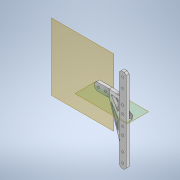
# Autodesk Inventor part: body_linker_2_8d
Saved by Autodesk Inventor 2023 (Build 270158000, 158)
## iProperties
Created: 2021-03-15
Part Number: body_linker_2_8d
Material: Generic
Document SubType Name: Modeling
Designer: Shuang Peng
Density: 1 g/cm^3
Appearance: Default
Author: Shuang Peng
Autodesk Inventor part; units mm, degrees
ref_plane "YZ Plane" through (0, 0, 0) normal (1, 0, 0) x (0, 1, 0)
ref_plane "XZ Plane" through (0, 0, 0) normal (0, 1, 0) x (-1, 0, 0)
ref_plane "XY Plane" through (0, 0, 0) normal (0, 0, 1) x (1, 0, 0)
sketch "Sketch1" plane through (0, 0, 0) normal (0, 0, 1) x (1, 0, 0)
  circle A0 centre (-13.3324, -4) radius 1.6 projected
  circle A1 centre (-13.3324, -14) radius 1.6 projected
  line L0 (-25.6648, -6) -> (-20.718, -6) projected
  arc A2 (-19.718, -7) -> (-20.718, -6) centre (-20.718, -7) ccw projected
  line L1 (-19.718, -7) -> (-19.718, -11) projected
  arc A3 (-20.718, -12) -> (-19.718, -11) centre (-20.718, -11) ccw projected
  line L2 (-20.718, -12) -> (-25.6648, -12) projected
  arc A4 (-26.6648, -11) -> (-25.6648, -12) centre (-25.6648, -11) ccw projected
  line L3 (-26.6648, -11) -> (-26.6648, -19) projected
  line L4 (-26.6648, -19) -> (0, -19) projected
  line L5 (0, -11) -> (0, -19) projected
  arc A5 (-1, -12) -> (0, -11) centre (-1, -11) ccw projected
  line L6 (-1, -12) -> (-5.9469, -12) projected
  arc A6 (-6.9469, -11) -> (-5.9469, -12) centre (-5.9469, -11) ccw projected
  line L7 (-6.9469, -11) -> (-6.9469, -7) projected
  arc A7 (-5.9469, -6) -> (-6.9469, -7) centre (-5.9469, -7) ccw projected
  line L8 (-5.9469, -6) -> (-1, -6) projected
  arc A8 (0, -7) -> (-1, -6) centre (-1, -7) ccw projected
  line L9 (0, 1) -> (0, -7) projected
  line L10 (-26.6648, 1) -> (0, 1) projected
  line L11 (-26.6648, 1) -> (-26.6648, -7) projected
  arc A9 (-25.6648, -6) -> (-26.6648, -7) centre (-25.6648, -7) ccw projected
  circle A10 centre (-13.3324, 53) radius 1.6 projected
  circle A11 centre (-13.3324, 63) radius 1.6 projected
  line L12 (-25.6648, 55) -> (-20.718, 55) projected
  arc A12 (-26.6648, 56) -> (-25.6648, 55) centre (-25.6648, 56) ccw projected
  line L13 (-26.6648, 48) -> (-26.6648, 56) projected
  line L14 (-26.6648, 48) -> (0, 48) projected
  line L15 (0, 48) -> (0, 56) projected
  arc A13 (-1, 55) -> (0, 56) centre (-1, 56) ccw projected
  line L16 (-5.9469, 55) -> (-1, 55) projected
  arc A14 (-6.9469, 56) -> (-5.9469, 55) centre (-5.9469, 56) ccw projected
  line L17 (-6.9469, 60) -> (-6.9469, 56) projected
  arc A15 (-5.9469, 61) -> (-6.9469, 60) centre (-5.9469, 60) ccw projected
  line L18 (-1, 61) -> (-5.9469, 61) projected
  arc A16 (0, 60) -> (-1, 61) centre (-1, 60) ccw projected
  line L19 (0, 60) -> (0, 68) projected
  line L20 (-26.6648, 68) -> (0, 68) projected
  line L21 (-26.6648, 60) -> (-26.6648, 68) projected
  arc A17 (-25.6648, 61) -> (-26.6648, 60) centre (-25.6648, 60) ccw projected
  line L22 (-20.718, 61) -> (-25.6648, 61) projected
  arc A18 (-19.718, 60) -> (-20.718, 61) centre (-20.718, 60) ccw projected
  line L23 (-19.718, 56) -> (-19.718, 60) projected
  arc A19 (-20.718, 55) -> (-19.718, 56) centre (-20.718, 56) ccw projected
  line L24 (-13.3324, 53) -> (-13.3324, -4)
  line L25 (-9.8324, -19) -> (-16.8324, -19)
  line L26 (-16.8324, -19) -> (-16.8324, 68)
  line L27 (-16.8324, 68) -> (-9.8324, 68)
  line L28 (-9.8324, 68) -> (-9.8324, -19)
  line L29 (-9.8324, -19) -> (-16.8324, 68) construction
  line L30 (-16.8324, -19) -> (-9.8324, 68) construction
  circle A20 centre (-13.3324, -14) radius 1
  circle A21 centre (-13.3324, -4) radius 1
  circle A22 centre (-13.3324, 53) radius 1
  circle A23 centre (-13.3324, 63) radius 1
  point P0 (0, 0)
  point P1 (-13.3324, 24.5)
  dimension "d0" = 7
  dimension "d1" = 87
  dimension "d2" = 2
  dimension "d3" = 2
  dimension "d4" = 2
  dimension "d5" = 2
  constraints: 14 end point, 4 centre point, 4 coincident, 3 midpoint, 2 parallel, 1 horizontal, 1 perpendicular, 1 vertical
  measures "d0" distance of L25.start L25.end
  measures "d1" distance of L25.end L26.end
  measures "d2" diameter of A20
  measures "d3" diameter of A21
  measures "d4" diameter of A22
  measures "d5" diameter of A23
extrude "Extrusion1" add sketch "Sketch1" along normal blind 3 contours A0 | A1 | L26 L14 L24 L10 | L10 L28 L4 L26 | L24 L14 L28 L10 | L26 L20 L28 L14 | A10 | A11
ref_plane "Work Plane1" through (-45.4275, 48, -16.9065) normal (0, 0, 1) x (1, 0, 0)
ref_plane "Work Plane2" through (-45.4275, 48, -16.9065) normal (0, 0, 1) x (1, 0, 0)
sketch "Sketch2" plane through (-45.4275, 48, -16.9065) normal (0, 0, 1) x (1, 0, 0)
  circle A0 centre (-48.7456, -23.5) radius 1.5 projected
  circle A1 centre (-9.8354, -23.5) radius 1.5 projected
  circle A2 centre (-55.7456, -23.5) radius 1.5 projected
  circle A3 centre (-2.8354, -23.5) radius 1.5 projected
  line L0 (0, 8) -> (0, -55) projected
  line L1 (0, 8) -> (-2.7967, 8) projected
  line L2 (-2.7967, 8) -> (-15.1567, 2.005) projected
  arc A4 (-23.8848, 0) -> (-15.1567, 2.005) centre (-23.8848, 20) ccw projected
  line L3 (-23.8848, 0) -> (-34.6962, 0) projected
  arc A5 (-43.4243, 2.005) -> (-34.6962, 0) centre (-34.6962, 20) ccw projected
  line L4 (-43.4243, 2.005) -> (-55.7843, 8) projected
  line L5 (-55.7843, 8) -> (-58.581, 8) projected
  line L6 (-58.581, 8) -> (-58.581, -55) projected
  line L7 (-58.581, -55) -> (-55.7843, -55) projected
  line L8 (-55.7843, -55) -> (-43.4243, -49.005) projected
  arc A6 (-34.6962, -47) -> (-43.4243, -49.005) centre (-34.6962, -67) ccw projected
  line L9 (-23.8848, -47) -> (-34.6962, -47) projected
  arc A7 (-15.1567, -49.005) -> (-23.8848, -47) centre (-23.8848, -67) ccw projected
  line L10 (-15.1567, -49.005) -> (-2.7967, -55) projected
  line L11 (-2.7967, -55) -> (0, -55) projected
  line L12 (-2.8354, -23.5) -> (-9.8354, -23.5)
  line L13 (-13.8354, -27.5) -> (-13.8354, -19.5)
  line L14 (-13.8354, -19.5) -> (1.1646, -19.5)
  line L15 (1.1646, -19.5) -> (1.1646, -27.5)
  line L16 (1.1646, -27.5) -> (-13.8354, -27.5)
  line L17 (-13.8354, -27.5) -> (1.1646, -19.5) construction
  line L18 (-13.8354, -19.5) -> (1.1646, -27.5) construction
  circle A8 centre (-2.8354, -23.5) radius 1
  circle A9 centre (-9.8354, -23.5) radius 1
  circle A10 centre (-36.7456, -23.5) radius 1.5 projected
  circle A11 centre (-21.8354, -23.5) radius 1.5 projected
  line L19 (-18.1506, -17.698) -> (-8.4396, -10.4664) projected
  arc A12 (-6.5914, -10.1803) -> (-8.4396, -10.4664) centre (-7.2451, -12.0705) ccw projected
  line L20 (-6.5914, -10.1803) -> (-4.1818, -11.0136) projected
  arc A13 (-2.8354, -12.9037) -> (-4.1818, -11.0136) centre (-4.8354, -12.9037) ccw projected
  line L21 (-2.8354, -12.9037) -> (-2.8354, -17.5) projected
  arc A14 (-4.8354, -19.5) -> (-2.8354, -17.5) centre (-4.8354, -17.5) ccw projected
  line L22 (-4.8354, -19.5) -> (-17.5533, -19.5) projected
  arc A15 (-18.1506, -17.698) -> (-17.5533, -19.5) centre (-17.5533, -18.5) ccw projected
  line L23 (-50.1414, -10.4664) -> (-40.4304, -17.698) projected
  arc A16 (-41.0277, -19.5) -> (-40.4304, -17.698) centre (-41.0277, -18.5) ccw projected
  line L24 (-41.0277, -19.5) -> (-53.7456, -19.5) projected
  arc A17 (-55.7456, -17.5) -> (-53.7456, -19.5) centre (-53.7456, -17.5) ccw projected
  line L25 (-55.7456, -17.5) -> (-55.7456, -12.9037) projected
  arc A18 (-54.3992, -11.0136) -> (-55.7456, -12.9037) centre (-53.7456, -12.9037) ccw projected
  line L26 (-54.3992, -11.0136) -> (-51.9896, -10.1803) projected
  arc A19 (-50.1414, -10.4664) -> (-51.9896, -10.1803) centre (-51.3359, -12.0705) ccw projected
  line L27 (-8.4396, -36.5336) -> (-18.1506, -29.302) projected
  arc A20 (-17.5533, -27.5) -> (-18.1506, -29.302) centre (-17.5533, -28.5) ccw projected
  line L28 (-17.5533, -27.5) -> (-4.8354, -27.5) projected
  arc A21 (-2.8354, -29.5) -> (-4.8354, -27.5) centre (-4.8354, -29.5) ccw projected
  line L29 (-2.8354, -29.5) -> (-2.8354, -34.0963) projected
  arc A22 (-4.1818, -35.9864) -> (-2.8354, -34.0963) centre (-4.8354, -34.0963) ccw projected
  line L30 (-4.1818, -35.9864) -> (-6.5914, -36.8197) projected
  arc A23 (-8.4396, -36.5336) -> (-6.5914, -36.8197) centre (-7.2451, -34.9295) ccw projected
  line L31 (-40.4304, -29.302) -> (-50.1414, -36.5336) projected
  arc A24 (-51.9896, -36.8197) -> (-50.1414, -36.5336) centre (-51.3359, -34.9295) ccw projected
  line L32 (-51.9896, -36.8197) -> (-54.3992, -35.9864) projected
  arc A25 (-55.7456, -34.0963) -> (-54.3992, -35.9864) centre (-53.7456, -34.0963) ccw projected
  line L33 (-55.7456, -34.0963) -> (-55.7456, -29.5) projected
  arc A26 (-53.7456, -27.5) -> (-55.7456, -29.5) centre (-53.7456, -29.5) ccw projected
  line L34 (-53.7456, -27.5) -> (-41.0277, -27.5) projected
  arc A27 (-40.4304, -29.302) -> (-41.0277, -27.5) centre (-41.0277, -28.5) ccw projected
  arc A28 (-11.559, -7.802) -> (-12.1562, -6) centre (-12.1562, -7) ccw projected
  line L35 (-11.559, -7.802) -> (-28.096, -20.1168) projected
  arc A29 (-30.485, -20.1168) -> (-28.096, -20.1168) centre (-29.2905, -18.5127) ccw projected
  line L36 (-30.485, -20.1168) -> (-47.022, -7.802) projected
  arc A30 (-46.4248, -6) -> (-47.022, -7.802) centre (-46.4248, -7) ccw projected
  line L37 (-46.4248, -6) -> (-12.1562, -6) projected
  arc A31 (-12.1562, -41) -> (-11.559, -39.198) centre (-12.1562, -40) ccw projected
  line L38 (-12.1562, -41) -> (-46.4248, -41) projected
  arc A32 (-47.022, -39.198) -> (-46.4248, -41) centre (-46.4248, -40) ccw projected
  line L39 (-47.022, -39.198) -> (-30.485, -26.8832) projected
  arc A33 (-28.096, -26.8832) -> (-30.485, -26.8832) centre (-29.2905, -28.4873) ccw projected
  line L40 (-28.096, -26.8832) -> (-11.559, -39.198) projected
  circle A34 centre (-52.7905, -6) radius 1.5 projected
  circle A35 centre (-5.7905, -6) radius 1.5 projected
  circle A36 centre (-52.7905, -41) radius 1.5 projected
  circle A37 centre (-5.7905, -41) radius 1.5 projected
  point P0 (45.4275, -48)
  point P1 (-6.3354, -23.5)
  dimension "d8" = 8
  dimension "d9" = 15
  dimension "d10" = 2
  dimension "d11" = 2
  constraints: 14 end point, 3 midpoint, 2 centre point, 2 coincident, 2 parallel, 1 horizontal, 1 perpendicular, 1 vertical
  measures "d8" distance of L13.start L13.end
  measures "d9" distance of L13.end L14.end
  measures "d10" diameter of A8
  measures "d11" diameter of A9
extrude "Extrusion2" add sketch "Sketch2" along normal blind 3 contours A1 | A3 | L14 L15 L16 L0 | L0 L16 L13 L14
sketch "Sketch3" plane through (-16.8324, -19, 0) normal (-1, 0, 0) x (0, 0, 1)
  line L0 (0, 87) -> (0, 0) projected
  line L1 (0, 0) -> (3, 0) projected
  line L2 (3, 87) -> (3, 0) projected
  line L3 (0, 87) -> (3, 87) projected
  line L4 (0, 87) -> (0, 0) projected
  line L5 (0, 43.5) -> (3, 43.5)
  line L6 (3, 43.5) -> (0, 43.5)
  line L7 (0, 43.5) -> (0, 23.5)
  line L8 (0, 23.5) -> (3, 23.5)
  line L9 (3, 23.5) -> (3, 43.5)
  line L10 (0, 43.5) -> (3, 43.5)
  line L11 (3, 43.5) -> (3, 63.5)
  line L12 (3, 63.5) -> (0, 63.5)
  line L13 (0, 63.5) -> (0, 43.5)
  point P0 (0, 19)
  dimension "d14" = 3
  dimension "d15" = 20
  dimension "d16" = 3
  dimension "d17" = 20
  constraints: 18 end point, 4 parallel, 2 horizontal, 2 midpoint, 2 perpendicular
  measures "d14" distance of L8.end L7.end
  measures "d15" distance of L7.end L6.end
  measures "d16" distance of L12.end L11.end
  measures "d17" distance of L11.end L10.end
loft "Loft1" add profiles "Sketch3" section 2 edges at (-44.2629, 24.5, -16.9065) (-44.2629, 28.5, -15.4065) (-44.2629, 24.5, -13.9065) (-44.2629, 20.5, -15.4065) contours L12 L2 L5 L0 | L5 L2 L8 L0
ref_plane "Work Plane3" through (-59.2629, 24.5, -16.9065) normal (0, -1, 0) x (1, 0, 0)
sketch "Sketch5" plane through (-59.2629, 24.5, -16.9065) normal (0, -1, 0) x (1, 0, 0)
  line L0 (42.4305, 19.9065) -> (42.4305, 16.9065) projected
  line L1 (42.4305, 19.9065) -> (15, 3) projected
  line L2 (15, 0) -> (15, 3) projected
  line L3 (42.4305, 16.9065) -> (15, 0) projected
  line L4 (42.4305, 16.9065) -> (49.4305, 16.9065) projected
  line L5 (49.4305, 16.9065) -> (49.4305, 19.9065) projected
  line L6 (42.4305, 19.9065) -> (49.4305, 19.9065) projected
  line L7 (42.4305, 16.9065) -> (42.4305, 19.9065) projected
  line L8 (49.4305, 16.9065) -> (49.4305, 11.9065)
  line L9 (49.4305, 11.9065) -> (15, 0)
  point P0 (59.2629, 16.9065)
  point P1 (42.4305, 16.9065)
  dimension "d22" = 5
  constraints: 4 end point, 1 vertical
  measures "d22" distance of L4.end L8.end
extrude "Extrusion3" add sketch "Sketch5" against normal mid plane 2 contours L4 L8 L9 L3
fillet "Fillet1" radius 3 1 edges at (-9.8324, 24.5, -5)
sketch "Sketch6" plane through (-16.8324, 25.5, 0) normal (0.5246872, 0, -0.8512951) x (-0.8512951, 0, -0.5246872)
  line L0 (0, 0) -> (32.222, 0) projected
  line L1 (32.222, 0) -> (32.222, 3) projected
  line L2 (0, 19) -> (32.222, 3) projected
  line L3 (0, 19) -> (0, 0) projected
  line L4 (32.222, -2) -> (0, -2) projected
  line L5 (0, -2) -> (0, -21) projected
  line L6 (0, -21) -> (32.222, -5) projected
  line L7 (32.222, -5) -> (32.222, -2) projected
  line L8 (2, 13.5409) -> (2, 2)
  line L9 (2, 2) -> (25.242, 2)
  line L10 (25.242, 2) -> (2, 13.5409)
  line L11 (2, -4) -> (2, -15.5409)
  line L12 (2, -15.5409) -> (25.242, -4)
  line L13 (25.242, -4) -> (2, -4)
  line L14 (-1.25, 0) -> (32.222, 0) projected
  line L15 (32.222, -2) -> (-1.25, -2) projected
  point P0 (-14.3294, -25.5)
  dimension "d26" = 2
  dimension "d27" = 2
  dimension "d28" = 4
  dimension "d29" = 4
  dimension "d30" = 2
  dimension "d31" = 2
  constraints: 12 end point, 6 parallel, 1 horizontal
  measures "d26" distance between parallel lines of L3 L8
  measures "d27" distance between parallel lines of L14 L9
  measures "d28" distance between parallel lines of L2 L10
  measures "d29" distance between parallel lines of L6 L12
  measures "d30" distance between parallel lines of L4 L13
  measures "d31" distance between parallel lines of L5 L11
extrude "Extrusion4" cut sketch "Sketch6" against normal blind 3 contours L10 L9 L8 | L13 L12 L11
fillet "Fillet2" radius 0.5 2 edges at (-38.9908, 27.5, -12.1571) (-38.9908, 21.5, -12.1571)
fillet "Fillet2" radius 1 2 edges at (-19.205, 39.0409, 0.0377) (-19.205, 9.9591, 0.0377)
fillet "Fillet2" radius 1.5 2 edges at (-19.205, 27.5, 0.0377) (-19.205, 21.5, 0.0377)
fillet "Fillet3" radius 3 2 edges at (-16.8324, 44.5, 1.5) (-16.8324, 4.5, 1.5)
chamfer "Chamfer1" distance 2 angle 45 4 edges at (-16.8324, 68, 1.5) (-9.8324, 68, 1.5) (-16.8324, -19, 1.5) (-9.8324, -19, 1.5)
chamfer "Chamfer2" distance 2 angle 45 2 edges at (-59.2629, 20.5, -15.4065) (-59.2629, 28.5, -15.4065)
sketch "Sketch7" plane through (0, 0, 0) normal (0, 0, -1) x (-1, 0, 0)
  line L0 (11.8324, -19) -> (9.8324, -17) projected
  line L1 (14.8324, -19) -> (11.8324, -19) projected
  line L2 (16.8324, -17) -> (14.8324, -19) projected
  line L3 (16.8324, 2.7768) -> (16.8324, -17) projected
  line L4 (16.8324, 23.5) -> (16.8324, 2.7768) projected
  line L5 (16.8324, 23.5) -> (9.8324, 23.5) projected
  line L6 (9.8324, -17) -> (9.8324, 23.5) projected
  circle A0 centre (13.3324, -4) radius 1 projected
  circle A1 centre (13.3324, -14) radius 1 projected
  circle A2 centre (13.3324, 53) radius 1 projected
  circle A3 centre (13.3324, 63) radius 1 projected
  line L7 (9.8324, 66) -> (11.8324, 68) projected
  line L8 (9.8324, 25.5) -> (9.8324, 66) projected
  line L9 (9.8324, 25.5) -> (16.8324, 25.5) projected
  line L10 (16.8324, 46.2232) -> (16.8324, 25.5) projected
  line L11 (16.8324, 66) -> (16.8324, 46.2232) projected
  line L12 (14.8324, 68) -> (16.8324, 66) projected
  line L13 (11.8324, 68) -> (14.8324, 68) projected
  line L14 (16.8324, 23.5) -> (9.8324, 23.5)
  circle A4 centre (13.3324, -4) radius 1 projected
  line L15 (13.3324, -4) -> (13.3324, 11)
  line L16 (13.3324, 11) -> (13.3324, 19)
  circle A5 centre (13.3324, 53) radius 1 projected
  line L17 (13.3324, 53) -> (13.3324, 38)
  line L18 (13.3324, 38) -> (13.3324, 30)
  circle A6 centre (13.3324, 11) radius 1
  circle A7 centre (13.3324, 19) radius 1
  circle A8 centre (13.3324, 30) radius 1
  circle A9 centre (13.3324, 38) radius 1
  point P0 (0, 0)
  dimension "d44" = 15
  dimension "d45" = 8
  dimension "d46" = 15
  dimension "d47" = 8
  dimension "d48" = 2
  dimension "d49" = 2
  dimension "d50" = 2
  dimension "d51" = 2
  constraints: 10 end point, 4 centre point, 4 coincident, 3 vertical, 1 collinear, 1 point on line
  measures "d44" distance of L15.start L15.end
  measures "d45" distance of L15.end L16.end
  measures "d46" distance of L17.start L17.end
  measures "d47" distance of L17.end L18.end
  measures "d48" diameter of A6
  measures "d49" diameter of A7
  measures "d50" diameter of A8
  measures "d51" diameter of A9
extrude "Extrusion5" cut sketch "Sketch7" against normal blind 3 contours A6 L16 L15 | L15 L16 A6 | A9 L18 L17 | L17 L18 A9 | A7 | A8
fillet "Fillet4" radius 1 4 edges at (-30.5477, 23.5, -8.4532) (-30.5477, 25.5, -8.4532) (-13.3324, 25.5, 0) (-13.3324, 23.5, 0)
body "Solid1"
